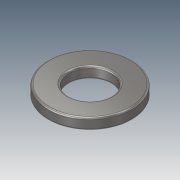
# Autodesk Inventor part: 900-80-WASHERS-ISO8738-8
Saved by Autodesk Inventor 2018.2 (Build 222227000, 227)
## iProperties
Manager: feesmrt
Company: FRANC0R
Created: 2017-12-05
Part Number: 900-80-WASHERS-ISO8738-8
Material: Edelstahl
Document SubType Name: Modeling
Designer: feesmrt
Density: 8 g/cm^3
Appearance: Halbpoliert
Project: Rescue Robot
Cost Center: -
Engineer: feesmrt
Authority: feesmrt
Description: Scheibe ISO 8738-8
Stock Number: 900-80-WASHERS-ISO8738-8
Author: feesmrt
Subject: Rescue Robot
Title: Scheibe ISO 8738-8
Revision Number: 1
Autodesk Inventor part; units mm, degrees
ref_plane "YZ Plane" through (0, 0, 0) normal (1, 0, 0) x (0, 1, 0)
ref_plane "XZ Plane" through (0, 0, 0) normal (0, 1, 0) x (-1, 0, 0)
ref_plane "XY Plane" through (0, 0, 0) normal (0, 0, 1) x (1, 0, 0)
sketch "Skizze1" plane through (0, 0, 0) normal (0, 0, 1) x (1, 0, 0)
  circle A0 centre (0, 0) radius 3
  circle A1 centre (0, 0) radius 6
  dimension "d0" = 6
  dimension "d1" = 12
  constraints: 2 centre point, 2 coincident
  measures "d0" diameter of A0
  measures "d1" diameter of A1
extrude "Extrusion1" add sketch "Skizze1" along normal mid plane 1.6
fillet "Rundung1" radius 0.25 4 edges at (-6, 0, 0.8) (-6, 0, -0.8) (-3, 0, 0.8) (-3, 0, -0.8)
